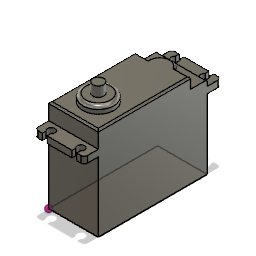
Hitec_HS-805MG (Autodesk Fusion 360 design; units mm, degrees)
Autodesk Fusion 360 part; units mm, degrees
sketch "Skizze1" plane through (0, 0, 0) normal (0, 1, 0) x (1, 0, 0)
  line L0 (0, 0) -> (30, 0)
  line L1 (30, 0) -> (30, 66)
  line L2 (30, 66) -> (0, 66)
  line L3 (0, 66) -> (0, 0)
  dimension "d5" = 30
  dimension "d6" = 66
  measures "d5" distance of L0.start L0.end
  measures "d6" distance of L0.start L2.end
extrude "Extrusion2" add sketch "Skizze1" along normal blind 42.2
sketch "Skizze2" plane through (0, 42.2, 0) normal (0, 1, 0) x (-1, 0, 0)
  line L0 (0, -66) -> (0, 0)
  line L1 (0, 0) -> (-30, 0)
  line L2 (-30, 0) -> (-30, -66)
  line L3 (-30, -66) -> (0, -66)
  line L4 (0, -74.5) -> (-30, -74.5)
  line L5 (-30, -74.5) -> (-30, 8.5)
  line L6 (-30, 8.5) -> (0, 8.5)
  line L7 (0, 8.5) -> (0, -74.5)
  line L8 (-30, -66) -> (0, 0) construction
  line L9 (0, -74.5) -> (-30, 8.5) construction
  line L10 (-15, -33) -> (-15, -70.5) construction
  line L11 (-15, -70.5) -> (-6, -70.5) construction
  circle A0 centre (-6, -70.5) radius 2.25
  circle A1 centre (-24, -70.5) radius 2.25
  circle A2 centre (-6, 4.5) radius 2.25
  circle A3 centre (-24, 4.5) radius 2.25
  line L12 (-4.6, -74.5) -> (-7.4, -74.5)
  line L13 (-7.4, -74.5) -> (-7.4, -71.5)
  line L14 (-7.4, -71.5) -> (-4.6, -71.5)
  line L15 (-4.6, -71.5) -> (-4.6, -74.5)
  line L16 (-6, -71.5) -> (-6, -70.5) construction
  line L17 (-25.4, -74.5) -> (-25.4, -71.5)
  line L18 (-22.6, -74.5) -> (-25.4, -74.5)
  line L19 (-22.6, -71.5) -> (-22.6, -74.5)
  line L20 (-25.4, -71.5) -> (-22.6, -71.5)
  line L21 (-7.4, 5.5) -> (-7.4, 8.5)
  line L22 (-4.6, 5.5) -> (-7.4, 5.5)
  line L23 (-4.6, 8.5) -> (-4.6, 5.5)
  line L24 (-7.4, 8.5) -> (-4.6, 8.5)
  line L25 (-25.4, 5.5) -> (-25.4, 8.5)
  line L26 (-22.6, 5.5) -> (-25.4, 5.5)
  line L27 (-22.6, 8.5) -> (-22.6, 5.5)
  line L28 (-25.4, 8.5) -> (-22.6, 8.5)
  point P0 (-15, -33)
  dimension "d9" = 30
  dimension "d10" = 83
  dimension "d13" = 9
  dimension "d14" = 37.5
  dimension "d15" = 4.5
  dimension "d18" = -18
  dimension "d19" = 75
  dimension "d20" = 2.8
  dimension "d21" = 3
  dimension "d24" = -18
  dimension "d25" = 80
  measures "d9" distance of L4.start L4.end
  measures "d10" distance of L4.start L6.end
  measures "d13" distance of L10.end L11.end
  measures "d14" distance of P0 L10.end
  measures "d15" diameter of A0
  measures "d20" distance of L13.end L14.end
  measures "d21" distance of L12.end L13.end
extrude "Extrusion3" add sketch "Skizze2" along normal blind 4 contours L0 L1 L2 L3 L5 L7 | L3 L4 L5 L7 A0 A1 L13 L15 L17 L19 | L1 L5 L6 L7 A2 A3 L21 L23 L25 L27
sketch "Skizze3" plane through (0, 46.2, 0) normal (0, 1, 0) x (-1, 0, 0)
  line L0 (-7.4, 6.2614) -> (-7.4, 8.5)
  line L1 (-7.4, 8.5) -> (-22.6, 8.5)
  line L2 (-22.6, 8.5) -> (-22.6, 6.2614)
  arc A0 (-25.4, 6.2614) -> (-22.6, 6.2614) centre (-24, 4.5) ccw
  line L3 (-25.4, 6.2614) -> (-25.4, 8.5)
  line L4 (-25.4, 8.5) -> (-30, 8.5)
  line L5 (-30, 8.5) -> (-30, -74.5)
  line L6 (-30, -74.5) -> (-25.4, -74.5)
  line L7 (-25.4, -74.5) -> (-25.4, -72.2614)
  arc A1 (-22.6, -72.2614) -> (-25.4, -72.2614) centre (-24, -70.5) ccw
  line L8 (-22.6, -72.2614) -> (-22.6, -74.5)
  line L9 (-22.6, -74.5) -> (-7.4, -74.5)
  line L10 (-7.4, -74.5) -> (-7.4, -72.2614)
  arc A2 (-4.6, -72.2614) -> (-7.4, -72.2614) centre (-6, -70.5) ccw
  line L11 (-4.6, -72.2614) -> (-4.6, -74.5)
  line L12 (-4.6, -74.5) -> (0, -74.5)
  line L13 (0, -74.5) -> (0, 8.5)
  line L14 (0, 8.5) -> (-4.6, 8.5)
  line L15 (-4.6, 8.5) -> (-4.6, 6.2614)
  arc A3 (-7.4, 6.2614) -> (-4.6, 6.2614) centre (-6, 4.5) ccw
  line L16 (-30, -66) -> (0, -66)
  line L17 (0, 0) -> (-30, 0)
  line L18 (0, -66) -> (-30, -66)
  line L19 (-30, 0) -> (0, 0)
extrude "Extrusion4" add sketch "Skizze3" along normal blind 3.5 contours L5 L13 L16 L17 L18 L19
fillet "Abrundung1" radius 2 4 edges at (30, 44.2, -74.5) (0, 44.2, -74.5) (30, 44.2, 8.5) (0, 44.2, 8.5)
sketch "Skizze4" plane through (0, 49.7, 0) normal (0, 1, 0) x (-1, 0, 0)
  line L0 (0, -66) -> (0, 0)
  line L1 (0, 0) -> (-30, 0)
  line L2 (-30, 0) -> (-30, -66)
  line L3 (-30, -66) -> (0, -66)
  line L4 (-30, -66) -> (0, -66)
  line L5 (0, -66) -> (0, 0)
  line L6 (-30, 0) -> (-30, -66)
  line L7 (0, 0) -> (-30, 0)
  line L8 (0, -52.3857) -> (-7.8134, -52.3857)
  line L9 (-30, -55.8819) -> (-20.9697, -55.8819)
  arc A0 (-20.9697, -55.8819) -> (-7.8134, -52.3857) centre (-14.8561, -52.3857) ccw
  line L10 (-30, -66) -> (0, -66)
  line L11 (0, -66) -> (0, 0)
  line L12 (-30, 0) -> (-30, -66)
  dimension "d31" = 13.6143
  dimension "d32" = 10.1181
  dimension "d33" = 7.8134
  dimension "d35" = 9.0303
  measures "d31" distance of L8 L10
  measures "d32" distance of L9 L10
  measures "d33" distance of L8.end L11
  measures "d35" distance of L9.start L9.end
extrude "Extrusion5" add sketch "Skizze4" along normal blind 6.507 contours L0 L1 L2 L5 L6 L7 L8 L9 A0 L11 L12
sketch "Skizze5" plane through (0, 56.207, 0) normal (0, 1, 0) x (-1, 0, 0)
  line L0 (0, -52.3857) -> (0, 0)
  line L1 (0, 0) -> (-30, 0)
  line L2 (-30, 0) -> (-30, -55.8819)
  line L3 (-30, -55.8819) -> (-20.9697, -55.8819)
  arc A0 (-20.9697, -55.8819) -> (-7.8134, -52.3857) centre (-14.8561, -52.3857) ccw
  line L4 (-7.8134, -52.3857) -> (0, -52.3857)
  circle A1 centre (-15, -15) radius 9.4153
  line L5 (-30, 0) -> (-30, -66)
  line L6 (0, 0) -> (-30, 0)
  dimension "d39" = 15
  dimension "d40" = 15
  dimension "d41" = 18.8307
  measures "d39" distance of A1.centre L5
  measures "d40" distance of A1.centre L6
  measures "d41" diameter of A1
extrude "Extrusion6" add sketch "Skizze5" along normal blind 4.5 contours A1
sketch "Skizze6" plane through (0, 60.707, 0) normal (0, 1, 0) x (-1, 0, 0)
  circle A0 centre (-15, -15) radius 9.4153
  circle A1 centre (-15, -15) radius 9.4153
  circle A2 centre (-15, -15) radius 3.315
  dimension "d45" = 6.63
  measures "d45" diameter of A2
extrude "Extrusion7" add sketch "Skizze6" along normal blind 6 contours A2
fillet "Abrundung3" radius 2 1 edges at (23.7782, 60.707, -18.4047)
fillet "Abrundung2" radius 1 7 edges at (13.0473, 56.207, -59.1921) (3.9067, 56.207, -52.3857) (25.4848, 56.207, -55.8819) (15, 49.7, -66) (15, 56.207, 0) (30, 56.207, -27.9409) (0, 56.207, -26.1929)
equation "d13 = ( 18 / 2 ) * 1 mm"
equation "d14 = ( 75 / 2 ) * 1 mm"
